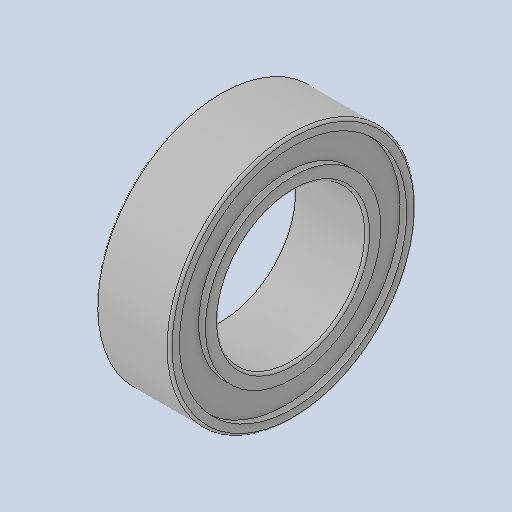
# Autodesk Inventor part: C-SE676ZZ
Saved by Autodesk Inventor 2024.1 (Build 281209000, 209)
## iProperties
Category: PARTsolutions
Company: MISUMI
Created: 2023-12-09
Part Number: C-SE676ZZ
Material: Generic
Catalog Web Link: www.cadenas.de
Description: C-SE___ZZ, C-SE___AZZ-Economy Stainless Miniature Deep Groove Ball Bearing - Double Shielded, Single Row
Vendor: MISUMI
Document SubType Name: Modeling
Designer: psAdmin
Manufacturer: MISUMI
Mass: 0.136063 g
Surface Area: 2.74665 cm^2
Volume: 0.136063 cm^3
Density: 1 g/cm^3
Appearance: PSOLRGB-175-175-175
PSOL_IDENT_0: {$CADENAS_DATA/23d-libs/misumi/metric/12_bearing_holders/c_se682zz.prj},173 {VTYP=3D},{NB=C-SE676ZZ}
PSOL_IDENT_1: ,{LINA=C-SE676ZZ},{NN=C-SE___ZZ, C-SE___AZZ},{DATE=29.05.2023 02:13:15},{GEOMDATE=25.05.2021 01:28:2
PSOL_IDENT_2: 4},{VERSION=},{LINEID=70},{WBVAR=},{WBNUMERIC=}  {NB=C-SE676ZZ},{LINA=C-SE676ZZ},{KT=DUMMY},{PN=C-SE
PSOL_IDENT_3: 676ZZ},{TS=C-SE676ZZ},{DD=6.0},{D=10},{B=3.0},{RR=0.10},{A=2.4600},{BB=0.400},{C=0.550}
NB: C-SE676ZZ
NN: C-SE___ZZ, C-SE___AZZ
NT: Economy Stainless Miniature Deep Groove Ball Bearing - Double Shielded, Single Row
NBSYN: $PN.
LINA: C-SE676ZZ
CATALOG: Misumi
PN: C-SE676ZZ
TS: C-SE676ZZ
DD: 6
D: 10
B: 3
RR: 0.1
SUPPLIER: MISUMI
ARTICLENO: C-SE676ZZ
BOMINFO: C-SE676ZZ
CREATOR: CADENAS GmbH
d1: 0.000 mm
Title: C-SE676ZZ
Author: Cadenas PARTsolutions
Comments: Economy Stainless Miniature Deep Groove Ball Bearing - Double Shielded, Single Row
Autodesk Inventor part; units mm, degrees
sketch "Sketch_1" plane through (0, 0, 0) normal (0, 0, 1) x (1, 0, 0)
  line L0 (2.9, 0) -> (0.1, 0)
  arc A0 (0, 3.1) -> (0.1, 3) centre (0.1, 3.1) ccw
  line L1 (0.1, 3) -> (2.9, 3)
  arc A1 (2.9, 3) -> (3, 3.1) centre (2.9, 3.1) ccw
  line L2 (3, 3.1) -> (3, 3.55)
  line L3 (3, 3.55) -> (2.73, 3.55)
  line L4 (2.73, 3.55) -> (2.73, 4.6)
  line L5 (2.73, 4.6) -> (3, 4.6)
  line L6 (3, 4.6) -> (3, 4.9)
  arc A2 (3, 4.9) -> (2.9, 5) centre (2.9, 4.9) ccw
  line L7 (2.9, 5) -> (0.1, 5)
  arc A3 (0.1, 5) -> (0, 4.9) centre (0.1, 4.9) ccw
  line L8 (0, 4.9) -> (0, 4.6)
  line L9 (0, 4.6) -> (0.27, 4.6)
  line L10 (0.27, 4.6) -> (0.27, 3.55)
  line L11 (0.27, 3.55) -> (0, 3.55)
  line L12 (0, 3.55) -> (0, 3.1)
  constraints: 26 end point, 8 point on circle, 4 centre point
revolve "Revolution1" add sketch "Sketch_1" angle 360 about axis through (2.9, 0, 0) along (1, 0, 0)
ref_plane "to_housing_XY" through (0, 0, 0) normal (1, 0, 0) x (0, 0, -1)
ref_plane "to_housing_YZ" through (0, 0, 0) normal (0, 0, -1) x (0, 1, 0)
ref_plane "to_housing_ZX" through (0, 0, 0) normal (0, 1, 0) x (1, 0, 0)
ref_plane "to_housing_center_XY" through (1.5, 0, 0) normal (1, 0, 0) x (0, 0, -1)
ref_plane "to_housing_center_YZ" through (1.5, 0, 0) normal (0, 0, -1) x (0, 1, 0)
ref_plane "to_housing_center_ZX" through (1.5, 0, 0) normal (0, 1, 0) x (1, 0, 0)
body "Solid1"
